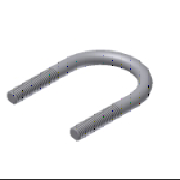
# Autodesk Inventor part: Скоба 40 ГОСТ 24137-80
Saved by Autodesk Inventor 2023 (Build 270158000, 158)
## iProperties
Created: 2022-02-04
Part Number: Скоба 40 ГОСТ 24137-80
Material: Сталь, мягкая
Description: Детали крепления трубопроводов. Скобы
Document SubType Name: Modeling
Standard: ГОСТ 24137-80
Designer: stepa
Standards Organization: GOST
Language: ru-RU
Size Designation: 40
Categories: <MemberInstance><Categories><Category DisplayName="Другие детали" InternalName="5aa15e00-363f-49f2-933f-16f664388e3f" Mnemonic="OTHER"><Category DisplayName="Соединения" InternalName="c83a05ef-9fc7-4930-b166-3bec2ee21d95" Mnemonic="LINKS"><CategoryParameter DisplayName="Ширина" InternalName="0146425d-1de7-4d10-87b7-50ac108f7d4d" Mnemonic="widthcl"/><CategoryParameter DisplayName="Длина" InternalName="b46efdc5-a45b-40d2-9b0b-cc8e7175b6f7" Mnemonic="lengthcl"/><CategoryParameter DisplayName="Номинальный диаметр" InternalName="e9ce5248-63ac-4968-a244-b114aebb38f3" Mnemonic="nomdia2"/><CategoryParameter DisplayName="Толщина" InternalName="eae647d9-8548-4b39-98cc-66a22ed53754" Mnemonic="thicknesscl"/></Category></Category><Category DisplayName="ТипДанных" InternalName="23b78d0f-2648-40c6-8793-ca6db495c9e8" Mnemonic="DATATYPE"><CategoryParameter DisplayName="ОтображаемоеИмя" InternalName="05415f3d-3907-474b-a020-eb9d644f4cf3" Mnemonic="DISPLAYNAME"/><CategoryParameter DisplayName="Стандарт" InternalName="0c0a119c-1e12-4c84-803f-101930972f5e" Mnemonic="STANDARD"/><CategoryParameter DisplayName="Наименование" InternalName="13903e3d-64b1-4950-80da-f627842ea37f" Mnemonic="DESCRIPTION"/><CategoryParameter DisplayName="Обозначение" InternalName="2675968c-4ce5-49e0-a4f5-552d29089031" Mnemonic="DESIGNATION"/><CategoryParameter DisplayName="Строка по умолчанию" InternalName="2af9ec52-faaa-4026-b378-f9fa4afca842" Mnemonic="DEFAULTROW"/><CategoryParameter DisplayName="Имя папки" InternalName="3f06958e-8713-4116-9be7-ed6184ecc97b" Mnemonic="FOLDERNAME"/><CategoryParameter DisplayName="Указатель редакций" InternalName="45a75005-10b1-4dfc-8d6d-dfe629f0b93c" Mnemonic="REVISIONGUID"/><CategoryParameter DisplayName="ИмяФайла" InternalName="8b46a4cc-9585-4fed-90c3-899f57e09a73" Mnemonic="FILENAME"/><CategoryParameter DisplayName="ОргСтанд" InternalName="8f5914e1-4693-403f-8ab5-d37768198c9d" Mnemonic="STDSORG"/><CategoryParameter DisplayName="Версия семейства" InternalName="914462f6-6e19-4b14-ba84-155b9680b1d0" Mnemonic="FAMILYREVISION"/><CategoryParameter DisplayName="Редакция стандарта" InternalName="91d5a463-65c2-4fde-b823-3b7fea5e8e17" Mnemonic="STANDARDREVISION"/><CategoryParameter DisplayName="редакция элемента" InternalName="a65d44b9-392f-4f4f-857b-e4b3d54996fe" Mnemonic="MEMBERREVISION"/><CategoryParameter DisplayName="ФорматКлипа" InternalName="bc51e27b-3422-4e78-93ef-cec197ddf230" Mnemonic="CLIPFORMAT"/><CategoryParameter DisplayName="Изготовитель" InternalName="cd6c7a72-a28a-4e50-99a9-2c7f4e13e5ad" Mnemonic="MANUFACTURER"/><CategoryParameter DisplayName="ВнутреннееИмя" InternalName="cf1d0246-76d9-4b4a-8305-fa0409afb5c1" Mnemonic="INTERNALNAME"/><CategoryParameter DisplayName="Метрическая" InternalName="e2385c5b-1ea4-4823-96a8-8de651266ec3" Mnemonic="ISMETRIC"/><Category DisplayName="Деталь" InternalName="c0e0b642-3bcb-4cc8-9e80-f96d35c4afa4" Mnemonic="PART"><CategoryParameter DisplayName="Номер детали" InternalName="016b6077-bfbe-49bd-92c9-d8d59c39c941" Mnemonic="PARTNUMBER"/><CategoryParameter DisplayName="Инвентарный номер" InternalName="4dba7c1c-e26c-444e-836c-b08b433409a8" Mnemonic="STOCKNUMBER"/><CategoryParameter DisplayName="Ключ материала" InternalName="5c9a8adb-dd2b-4535-b97f-0a94a95fe41f" Mnemonic="MATERIALKEY"/><CategoryParameter DisplayName="Материал" InternalName="818a152a-d3c3-49ca-80ee-df7d91421b8e" Mnemonic="MATERIAL"/></Category></Category></Categories><FamilyTemplate Id="Clamp GOST 24137-80"><FamilyTemplateParameters><FamilyTemplateParameter ObjectType="kUserParameterObject" ValueType="xs:double" Id="1" ObjectReferenceKey="A_"/><FamilyTemplateParameter ObjectType="kUserParameterObject" ValueType="xs:double" Id="2" ObjectReferenceKey="D"/><FamilyTemplateParameter ObjectType="kUserParameterObject" ValueType="xs:double" Id="3" ObjectReferenceKey="d_"/><FamilyTemplateParameter ObjectType="kUserParameterObject" ValueType="xs:double" Id="4" ObjectReferenceKey="H_"/><FamilyTemplateParameter ObjectType="kUserParameterObject" ValueType="xs:double" Id="5" ObjectReferenceKey="l_"/><FamilyTemplateParameter ObjectType="kPropertyObject" ValueType="xs:string" Id="100" ObjectReferenceKey="{32853F0F-3444-11d1-9E93-0060B03C1CA6}" SubObjectId="52"/><FamilyTemplateParameter ObjectType="kPropertyObject" ValueType="xs:string" Id="105" ObjectReferenceKey="{32853F0F-3444-11d1-9E93-0060B03C1CA6}" SubObjectId="5"/><FamilyTemplateParameter ObjectType="kPartComponentDefinitionObject" ValueType="xs:string" Id="110" SubObjectId="Material"/><FamilyTemplateParameter ObjectType="kThreadFeatureObject" ValueType="xs:structure" Id="300" ObjectReferenceKey="10020000100000008f010000000000008000000000000000" SubObjectId="ThreadInfo"><FamilyTemplateParameter ObjectType="" ValueType="xs:string" Id="301" SubObjectId="ThreadClass"/><FamilyTemplateParameter ObjectType="" ValueType="xs:string" Id="302" SubObjectId="ThreadDesignation"/><FamilyTemplateParameter ObjectType="" ValueType="xs:string" Id="303" SubObjectId="ThreadType"/></FamilyTemplateParameter><FamilyTemplateParameter ObjectType="kThreadFeatureObject" ValueType="xs:structure" Id="304" ObjectReferenceKey="1002000010000000b40a0000000000008000000000000000" SubObjectId="ThreadInfo"><FamilyTemplateParameter ObjectType="" ValueType="xs:string" Id="305" SubObjectId="ThreadClass"/><FamilyTemplateParameter ObjectType="" ValueType="xs:string" Id="306" SubObjectId="ThreadDesignation"/><FamilyTemplateParameter ObjectType="" ValueType="xs:string" Id="307" SubObjectId="ThreadType"/></FamilyTemplateParameter></FamilyTemplateParameters></FamilyTemplate><CategoryParameterMap><ParamToTemplateMap><ParamToTemplate CategoryParameter="//CategoryParameter[@InternalName='05415f3d-3907-474b-a020-eb9d644f4cf3']" ConstantValue="Clamp GOST 24137-80"/><ParamToTemplate CategoryParameter="//CategoryParameter[@InternalName='0c0a119c-1e12-4c84-803f-101930972f5e']" ConstantValue="GOST 24137-80"/><ParamToTemplate CategoryParameter="//CategoryParameter[@InternalName='13903e3d-64b1-4950-80da-f627842ea37f']" ConstantValue="Pipe-line fastening parts.Clamps"/><ParamToTemplate CategoryParameter="//CategoryParameter[@InternalName='2af9ec52-faaa-4026-b378-f9fa4afca842']" ConstantValue="1"/><ParamToTemplate CategoryParameter="//CategoryParameter[@InternalName='3f06958e-8713-4116-9be7-ed6184ecc97b']" ConstantValue="Clamp GOST 24137-80"/><ParamToTemplate CategoryParameter="//CategoryParameter[@InternalName='45a75005-10b1-4dfc-8d6d-dfe629f0b93c']" ConstantValue="5e28b2fa-667e-4e79-8e0c-9b77393244f8"/><ParamToTemplate CategoryParameter="//CategoryParameter[@InternalName='8f5914e1-4693-403f-8ab5-d37768198c9d']" ConstantValue="GOST"/><ParamToTemplate CategoryParameter="//CategoryParameter[@InternalName='914462f6-6e19-4b14-ba84-155b9680b1d0']" ConstantValue="11"/><ParamToTemplate CategoryParameter="//CategoryParameter[@InternalName='91d5a463-65c2-4fde-b823-3b7fea5e8e17']" TemplateParameter="103"/><ParamToTemplate CategoryParameter="//CategoryParameter[@InternalName='bc51e27b-3422-4e78-93ef-cec197ddf230']" ConstantValue="CF_INVENTOR.STDPARTS"/><ParamToTemplate CategoryParameter="//CategoryParameter[@InternalName='cd6c7a72-a28a-4e50-99a9-2c7f4e13e5ad']" TemplateParameter="104"/><ParamToTemplate CategoryParameter="//CategoryParameter[@InternalName='cf1d0246-76d9-4b4a-8305-fa0409afb5c1']" ConstantValue="0061bf7c-9b4c-4aab-ac10-bf23c251f687"/><ParamToTemplate CategoryParameter="//CategoryParameter[@InternalName='e2385c5b-1ea4-4823-96a8-8de651266ec3']" ConstantValue="true"/><ParamToTemplate CategoryParameter="//CategoryParameter[@InternalName='8b46a4cc-9585-4fed-90c3-899f57e09a73']" ConstantValue="Скоба 40 ГОСТ 24137-80"/><ParamToTemplate CategoryParameter="//CategoryParameter[@InternalName='a65d44b9-392f-4f4f-857b-e4b3d54996fe']" ConstantValue="47aca863-f0b2-4aad-aacd-4220840a1643"/><ParamToTemplate CategoryParameter="//CategoryParameter[@InternalName='e9ce5248-63ac-4968-a244-b114aebb38f3']" TemplateParameter="2"/><ParamToTemplate CategoryParameter="//CategoryParameter[@InternalName='2675968c-4ce5-49e0-a4f5-552d29089031']" TemplateParameter="100"/><ParamToTemplate CategoryParameter="//CategoryParameter[@InternalName='0146425d-1de7-4d10-87b7-50ac108f7d4d']" TemplateParameter="4"/><ParamToTemplate CategoryParameter="//CategoryParameter[@InternalName='818a152a-d3c3-49ca-80ee-df7d91421b8e']" TemplateParameter="110"/><ParamToTemplate CategoryParameter="//CategoryParameter[@InternalName='016b6077-bfbe-49bd-92c9-d8d59c39c941']" TemplateParameter="105"/></ParamToTemplateMap></CategoryParameterMap></MemberInstance>
Density: 7.85 g/cm^3
Appearance: С умеренной полировкой
IsCustomPart: 0
Title: Хомут
Author: stepa
Autodesk Inventor part; units mm, degrees
ref_plane "YZ Plane" through (0, 0, 0) normal (1, 0, 0) x (0, 1, 0)
ref_plane "XZ Plane" through (0, 0, 0) normal (0, 1, 0) x (-1, 0, 0)
sketch "Sketch1" plane through (0, 0, 0) normal (0, 0, 1) x (1, 0, 0)
  arc A0 (24, 0) -> (-24, 0) centre (0, 0) ccw
  line L0 (-24, 0) -> (-24, -44)
  line L1 (24, 0) -> (24, -44)
  dimension "d0" = 48
  dimension "d1" = 44
  constraints: 4 end point, 2 point on circle, 2 tangent, 1 centre point, 1 coincident, 1 horizontal alignment, 1 parallel, 1 vertical
  measures "d0" diameter of A0
  measures "d1" distance of L1.start L1.end
ref_plane "Work Plane1" through (-24, -44, 0) normal (0, -1, 0) x (1, 0, 0)
sketch "Sketch2" plane through (-24, -44, 0) normal (0, -1, 0) x (1, 0, 0)
  circle A0 centre (0, 0) radius 4
  point P0 (24, 0)
  dimension "d2" = 8
  constraints: 1 centre point
  measures "d2" diameter of A0
sweep "Колебание1" add profiles "Sketch2" path "Sketch1"
thread "Резьба1"
thread "Резьба2"
chamfer "Фаска1" distance 1 angle 45 2 edges at (28, -44, 0) (-28, -44, 0)
equation "\"d0\" = D + d_"
equation "\"d1\" = -d_ + H_ - 0.5 * D"
equation "\"d2\" = d_"
equation "\"d4\" = l_"
equation "\"d11\" = l_"
equation "\"D\" = 40"
equation "\"A_\" = 48"
equation "\"H_\" = 72"
equation "\"d_\" = 8"
equation "\"l_\" = 34"
body "Solid1"
